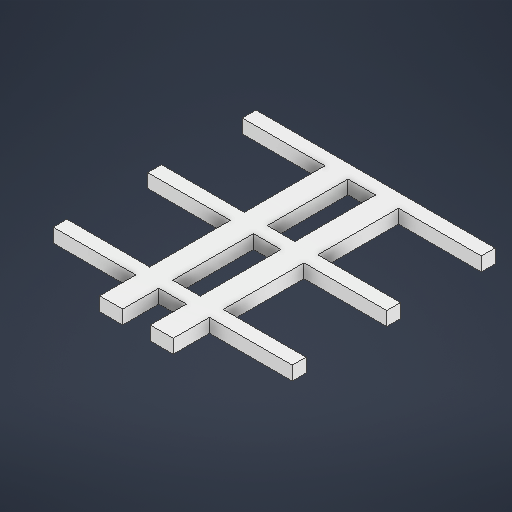
# Autodesk Inventor part: module-switch_port-catch
Saved by Autodesk Inventor 2025.2 (Build 292293000, 293)
## iProperties
Created: 2026-01-02
Part Number: module-switch_port-catch
Material: PC/ABS Plastic
Document SubType Name: Modeling
Designer: sam
Density: 1.1 g/cm^3
Appearance: Smooth - White
Author: sam
Autodesk Inventor part; units mm, degrees
ref_plane "YZ Plane" through (0, 0, 0) normal (1, 0, 0) x (0, 1, 0)
ref_plane "XZ Plane" through (0, 0, 0) normal (0, 1, 0) x (-1, 0, 0)
ref_plane "XY Plane" through (0, 0, 0) normal (0, 0, 1) x (1, 0, 0)
sketch "Sketch1" plane through (0, 0, 0) normal (0, 1, 0) x (-1, 0, 0)
  line L0 (0, 0) -> (-5, 0)
  line L1 (-5, 0) -> (-5, 50)
  line L2 (-5, 50) -> (0, 50)
  line L3 (0, 50) -> (0, 0)
  line L4 (-16, 50) -> (-11, 50)
  line L5 (-11, 50) -> (-11, 0)
  line L6 (-11, 0) -> (-16, 0)
  line L7 (-16, 0) -> (-16, 50)
  line L8 (18, 1) -> (-34, 1)
  line L9 (-34, 1) -> (-34, -2)
  line L10 (-34, -2) -> (18, -2)
  line L11 (18, -2) -> (18, 1)
  line L12 (-5, 0) -> (-11, 0)
  line L13 (18, 18.56) -> (-34, 18.56)
  line L14 (-34, 18.56) -> (-34, 21.56)
  line L15 (-34, 21.56) -> (18, 21.56)
  line L16 (18, 21.56) -> (18, 18.56)
  line L17 (18, 39.12) -> (-34, 39.12)
  line L18 (-34, 39.12) -> (-34, 42.12)
  line L19 (-34, 42.12) -> (18, 42.12)
  line L20 (18, 42.12) -> (18, 39.12)
  point P0 (-8, 0)
  point P1 (-8, -2)
  point P2 (0, 18.56)
  point P3 (0, 21.56)
  point P4 (0, 39.12)
  point P5 (0, 42.12)
  point P6 (-5, 42.12)
  point P7 (-11, 42.12)
  point P8 (-16, 42.12)
  point P9 (-16, 39.12)
  point P10 (-16, 21.56)
  point P11 (-16, 18.56)
  point P12 (-16, 1)
  point P13 (0, 1)
  point P14 (-11, 21.56)
  point P15 (-11, 39.12)
  point P16 (-5, 39.12)
  point P17 (-5, 21.56)
  point P18 (-5, 18.56)
  point P19 (-5, 1)
  point P20 (-11, 1)
  point P21 (-11, 18.56)
  point P22 (-8, 18.56)
  dimension "d0" = 5
  dimension "d1" = 50
  dimension "d3" = 5
  dimension "d4" = 50
  dimension "d5" = 52
  dimension "d6" = 3
  dimension "d7" = 1
  dimension "d8" = 0
  dimension "d9" = 52
  dimension "d10" = 3
  dimension "d11" = 52
  dimension "d12" = 3
  dimension "d16" = 20.56
  dimension "d17" = 20.56
  dimension "d20" = 16
  dimension "d21" = 0
  constraints: 42 end point, 10 parallel, 5 horizontal, 5 perpendicular, 3 midpoint, 1 collinear, 1 point on line
  measures "d0" distance of L1.end L2.end
  measures "d1" distance of L0.end L1.end
  measures "d3" distance between parallel lines of L7 L5
  measures "d4" distance between parallel lines of L4 L6
  measures "d5" distance of L10.end L9.end
  measures "d6" distance of L9.end L8.end
  measures "d7" distance between parallel lines of L6 L8
  measures "d8" horizontal distance of point (-8, 0) point (-8, -2)
  measures "d9" distance of L14.end L15.end
  measures "d10" distance of L13.end L14.end
  measures "d11" distance of L18.end L19.end
  measures "d12" distance of L17.end L18.end
  measures "d16" distance between parallel lines of L15 L8
  measures "d17" distance between parallel lines of L19 L15
  measures "d20" distance between parallel lines of L7 L3
  measures "d21" horizontal distance of point (-8, 0) point (-8, 18.56)
extrude "Extrusion1" add sketch "Sketch1" along normal blind 3 contours L3 L8 L11 L10 L9 L7 L6 L12 L0 | L0 L1 L8 L3 | L12 L5 L8 L1 | L8 L1 L13 L3 | L6 L7 L8 L5 | L13 L1 L15 L3 | L3 L15 L16 L13 | L13 L5 L15 L1 | L8 L7 L13 L5 | L15 L1 L17 L3 | L13 L7 L15 L5 | L17 L1 L19 L3 | L3 L19 L20 L17 | L17 L5 L19 L1 | L15 L7 L17 L5 | L13 L14 L15 L7 | L19 L1 L2 L3 | L17 L7 L19 L5 | L19 L7 L4 L5 | L17 L18 L19 L7
equation "\"d3\" = d0"
equation "\"d4\" = d1"
body "Solid1"
